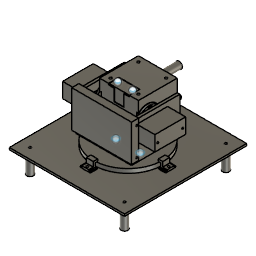
torretta_modulare_stampabile_v6_doppia_D_5x3x6 (Autodesk Fusion 360 design; units mm, degrees)
part number: 2026-07-14-16-52-52-233
part number: 2026-07-14-16-52-52-512
part number: 2026-07-14-16-52-55-927
part number: 2026-07-14-16-52-56-118
part number: 2026-07-14-16-52-56-486
part number: 2026-07-14-16-52-56-983
part number: 2026-07-14-16-52-59-861
part number: 2026-07-14-16-53-01-175
part number: 2026-07-14-16-53-03-719
part number: 2026-07-14-16-53-06-928
part number: 2026-07-14-16-53-10-286
part number: 2026-07-14-16-53-52-577
part number: 2026-07-14-16-53-58-816
part number: 2026-07-14-16-54-05-339
part number: 2026-07-14-16-54-28-797
part number: 2026-07-14-16-54-36-418
part number: 2026-07-14-16-54-44-458
part number: 2026-07-14-16-54-54-993
part number: 2026-07-14-16-55-05-930
part number: 2026-07-14-16-55-25-983
part number: 2026-07-14-16-55-55-201
part number: 2026-07-14-16-56-11-830
part number: 2026-07-14-16-56-28-975
part number: 2026-07-14-16-57-31-227
Autodesk Fusion 360 part; units mm, degrees
(part 1 of 3)
ref_plane "Piano di lavoro1" through (0, 0, 30) normal (0, 0, 1) x (1, 0, 0) in component "01_Tetto_elettronica_removibile"
sketch "Schizzo1" plane through (0, 0, 30) normal (0, 0, 1) x (1, 0, 0) in component "01_Tetto_elettronica_removibile"
  line L0 (-83, -88) -> (83, -88)
  line L1 (83, -88) -> (83, 88)
  line L2 (83, 88) -> (-83, 88)
  line L3 (-83, 88) -> (-83, -88)
extrude "Estrusione_Tetto_coperchio" add sketch "Schizzo1" along normal blind 3 makes body 1 in component "01_Tetto_elettronica_removibile"
sketch "Schizzo2" plane through (0, 0, 0) normal (0, 0, 1) x (1, 0, 0) in component "01_Tetto_elettronica_removibile"
  circle A0 centre (-68, -73) radius 5
extrude "Estrusione_Boss_verticale_M3_coperchio_01" add sketch "Schizzo2" along normal blind 33 bodies 1 in component "01_Tetto_elettronica_removibile"
sketch "Schizzo3" plane through (0, 0, 0) normal (0, 0, 1) x (1, 0, 0) in component "01_Tetto_elettronica_removibile"
  circle A0 centre (-68, -73) radius 1.6
extrude "Foro_M3_accessibile_dal_tetto_01" cut sketch "Schizzo3" along normal blind 33 bodies 1 in component "01_Tetto_elettronica_removibile"
sketch "Schizzo4" plane through (0, 0, 0) normal (0, 0, 1) x (1, 0, 0) in component "01_Tetto_elettronica_removibile"
  circle A0 centre (68, -73) radius 5
extrude "Estrusione_Boss_verticale_M3_coperchio_02" add sketch "Schizzo4" along normal blind 33 bodies 1 in component "01_Tetto_elettronica_removibile"
sketch "Schizzo5" plane through (0, 0, 0) normal (0, 0, 1) x (1, 0, 0) in component "01_Tetto_elettronica_removibile"
  circle A0 centre (68, -73) radius 1.6
extrude "Foro_M3_accessibile_dal_tetto_02" cut sketch "Schizzo5" along normal blind 33 bodies 1 in component "01_Tetto_elettronica_removibile"
sketch "Schizzo6" plane through (0, 0, 0) normal (0, 0, 1) x (1, 0, 0) in component "01_Tetto_elettronica_removibile"
  circle A0 centre (-68, 73) radius 5
extrude "Estrusione_Boss_verticale_M3_coperchio_03" add sketch "Schizzo6" along normal blind 33 bodies 1 in component "01_Tetto_elettronica_removibile"
sketch "Schizzo7" plane through (0, 0, 0) normal (0, 0, 1) x (1, 0, 0) in component "01_Tetto_elettronica_removibile"
  circle A0 centre (-68, 73) radius 1.6
extrude "Foro_M3_accessibile_dal_tetto_03" cut sketch "Schizzo7" along normal blind 33 bodies 1 in component "01_Tetto_elettronica_removibile"
sketch "Schizzo8" plane through (0, 0, 0) normal (0, 0, 1) x (1, 0, 0) in component "01_Tetto_elettronica_removibile"
  circle A0 centre (68, 73) radius 5
extrude "Estrusione_Boss_verticale_M3_coperchio_04" add sketch "Schizzo8" along normal blind 33 bodies 1 in component "01_Tetto_elettronica_removibile"
sketch "Schizzo9" plane through (0, 0, 0) normal (0, 0, 1) x (1, 0, 0) in component "01_Tetto_elettronica_removibile"
  circle A0 centre (68, 73) radius 1.6
extrude "Foro_M3_accessibile_dal_tetto_04" cut sketch "Schizzo9" along normal blind 33 bodies 1 in component "01_Tetto_elettronica_removibile"
ref_plane "Piano di lavoro2" through (0, 0, 30) normal (0, 0, 1) x (1, 0, 0) in component "01_Tetto_elettronica_removibile"
ref_plane "Piano di lavoro3" through (0, 0, 33) normal (0, 0, 1) x (1, 0, 0) in component "01_Tetto_elettronica_removibile"
ref_plane "Piano di lavoro4" through (0, 0, 30.9) normal (0, 0, 1) x (1, 0, 0) in component "01_Tetto_elettronica_removibile"
sketch "Schizzo10" plane through (0, 0, 30) normal (0, 0, 1) x (1, 0, 0) in component "01_Tetto_elettronica_removibile"
  circle A0 centre (0, 0) radius 6.25
extrude "Passaggio_albero_stepper" cut sketch "Schizzo10" along normal blind 3 bodies 1 in component "01_Tetto_elettronica_removibile"
sketch "Schizzo11" plane through (0, 0, 30) normal (0, 0, 1) x (1, 0, 0) in component "01_Tetto_elettronica_removibile"
  circle A0 centre (-17.5, 0) radius 2.1
extrude "Foro_stepper_Ovest" cut sketch "Schizzo11" along normal blind 3 bodies 1 in component "01_Tetto_elettronica_removibile"
sketch "Schizzo12" plane through (0, 0, 30.9) normal (0, 0, 1) x (1, 0, 0) in component "01_Tetto_elettronica_removibile"
  circle A0 centre (-17.5, 0) radius 2.1
sketch "Schizzo13" plane through (0, 0, 33) normal (0, 0, 1) x (1, 0, 0) in component "01_Tetto_elettronica_removibile"
  circle A0 centre (-17.5, 0) radius 4.2
loft "Svasatura_90_gradi_stepper_Ovest" cut profiles "Schizzo12", "Schizzo13" section 1 section 2 bodies 1 in component "01_Tetto_elettronica_removibile"
sketch "Schizzo14" plane through (0, 0, 30) normal (0, 0, 1) x (1, 0, 0) in component "01_Tetto_elettronica_removibile"
  circle A0 centre (17.5, 0) radius 2.1
extrude "Foro_stepper_Est" cut sketch "Schizzo14" along normal blind 3 bodies 1 in component "01_Tetto_elettronica_removibile"
sketch "Schizzo15" plane through (0, 0, 30.9) normal (0, 0, 1) x (1, 0, 0) in component "01_Tetto_elettronica_removibile"
  circle A0 centre (17.5, 0) radius 2.1
sketch "Schizzo16" plane through (0, 0, 33) normal (0, 0, 1) x (1, 0, 0) in component "01_Tetto_elettronica_removibile"
  circle A0 centre (17.5, 0) radius 4.2
loft "Svasatura_90_gradi_stepper_Est" cut profiles "Schizzo15", "Schizzo16" section 1 section 2 bodies 1 in component "01_Tetto_elettronica_removibile"
sketch "Schizzo17" plane through (0, 0, 30) normal (0, 0, 1) x (1, 0, 0) in component "01_Tetto_elettronica_removibile"
  circle A0 centre (58.5, 0) radius 1.6
extrude "Foro_M3_fermaglio_anti_sollevamento_Est" cut sketch "Schizzo17" along normal blind 3 bodies 1 in component "01_Tetto_elettronica_removibile"
sketch "Schizzo18" plane through (0, 0, 30) normal (0, 0, 1) x (1, 0, 0) in component "01_Tetto_elettronica_removibile"
  line L0 (61.4, 1.6743) -> (58.5, 3.3486)
  line L1 (58.5, 3.3486) -> (55.6, 1.6743)
  line L2 (55.6, 1.6743) -> (55.6, -1.6743)
  line L3 (55.6, -1.6743) -> (58.5, -3.3486)
  line L4 (58.5, -3.3486) -> (61.4, -1.6743)
  line L5 (61.4, -1.6743) -> (61.4, 1.6743)
extrude "Sede_dado_M3_fermaglio_Est" cut sketch "Schizzo18" along normal blind 2.6 bodies 1 in component "01_Tetto_elettronica_removibile"
sketch "Schizzo19" plane through (0, 0, 30) normal (0, 0, 1) x (1, 0, 0) in component "01_Tetto_elettronica_removibile"
  circle A0 centre (-58.5, 0) radius 1.6
extrude "Foro_M3_fermaglio_anti_sollevamento_Ovest" cut sketch "Schizzo19" along normal blind 3 bodies 1 in component "01_Tetto_elettronica_removibile"
sketch "Schizzo20" plane through (0, 0, 30) normal (0, 0, 1) x (1, 0, 0) in component "01_Tetto_elettronica_removibile"
  line L0 (-55.6, 1.6743) -> (-58.5, 3.3486)
  line L1 (-58.5, 3.3486) -> (-61.4, 1.6743)
  line L2 (-61.4, 1.6743) -> (-61.4, -1.6743)
  line L3 (-61.4, -1.6743) -> (-58.5, -3.3486)
  line L4 (-58.5, -3.3486) -> (-55.6, -1.6743)
  line L5 (-55.6, -1.6743) -> (-55.6, 1.6743)
extrude "Sede_dado_M3_fermaglio_Ovest" cut sketch "Schizzo20" along normal blind 2.6 bodies 1 in component "01_Tetto_elettronica_removibile"
sketch "Schizzo21" plane through (0, 0, 30) normal (0, 0, 1) x (1, 0, 0) in component "01_Tetto_elettronica_removibile"
  circle A0 centre (0, 58.5) radius 1.6
extrude "Foro_M3_fermaglio_anti_sollevamento_Nord" cut sketch "Schizzo21" along normal blind 3 bodies 1 in component "01_Tetto_elettronica_removibile"
sketch "Schizzo22" plane through (0, 0, 30) normal (0, 0, 1) x (1, 0, 0) in component "01_Tetto_elettronica_removibile"
  line L0 (2.9, 60.1743) -> (0, 61.8486)
  line L1 (0, 61.8486) -> (-2.9, 60.1743)
  line L2 (-2.9, 60.1743) -> (-2.9, 56.8257)
  line L3 (-2.9, 56.8257) -> (0, 55.1514)
  line L4 (0, 55.1514) -> (2.9, 56.8257)
  line L5 (2.9, 56.8257) -> (2.9, 60.1743)
extrude "Sede_dado_M3_fermaglio_Nord" cut sketch "Schizzo22" along normal blind 2.6 bodies 1 in component "01_Tetto_elettronica_removibile"
sketch "Schizzo23" plane through (0, 0, 30) normal (0, 0, 1) x (1, 0, 0) in component "01_Tetto_elettronica_removibile"
  circle A0 centre (0, -58.5) radius 1.6
extrude "Foro_M3_fermaglio_anti_sollevamento_Sud" cut sketch "Schizzo23" along normal blind 3 bodies 1 in component "01_Tetto_elettronica_removibile"
sketch "Schizzo24" plane through (0, 0, 30) normal (0, 0, 1) x (1, 0, 0) in component "01_Tetto_elettronica_removibile"
  line L0 (2.9, -56.8257) -> (0, -55.1514)
  line L1 (0, -55.1514) -> (-2.9, -56.8257)
  line L2 (-2.9, -56.8257) -> (-2.9, -60.1743)
  line L3 (-2.9, -60.1743) -> (0, -61.8486)
  line L4 (0, -61.8486) -> (2.9, -60.1743)
  line L5 (2.9, -60.1743) -> (2.9, -56.8257)
extrude "Sede_dado_M3_fermaglio_Sud" cut sketch "Schizzo24" along normal blind 2.6 bodies 1 in component "01_Tetto_elettronica_removibile"
ref_plane "Piano di lavoro5" through (0, 0, 22.8) normal (0, 0, 1) x (1, 0, 0) in component "01_Tetto_elettronica_removibile"
sketch "Schizzo25" plane through (0, 0, 22.8) normal (0, 0, 1) x (1, 0, 0) in component "01_Tetto_elettronica_removibile"
  circle A0 centre (0, 0) radius 23.5
  circle A1 centre (0, 0) radius 22
extrude "Estrusione_Parete_interna_liscia_canale_cavi" add sketch "Schizzo25" along normal blind 7.4 bodies 1 in component "01_Tetto_elettronica_removibile"
sketch "Schizzo26" plane through (0, 0, 22.8) normal (0, 0, 1) x (1, 0, 0) in component "01_Tetto_elettronica_removibile"
  circle A0 centre (0, 0) radius 34
  circle A1 centre (0, 0) radius 32.5
extrude "Estrusione_Parete_esterna_liscia_canale_cavi" add sketch "Schizzo26" along normal blind 7.4 bodies 1 in component "01_Tetto_elettronica_removibile"
ref_plane "Piano di lavoro6" through (0, 0, 20) normal (0, 0, 1) x (1, 0, 0) in component "01_Tetto_elettronica_removibile"
sketch "Schizzo27" plane through (0, 0, 20) normal (0, 0, 1) x (1, 0, 0) in component "01_Tetto_elettronica_removibile"
  circle A0 centre (0, 0) radius 40
  circle A1 centre (0, 0) radius 19
extrude "Estrusione_Fondo_anulare_continuo_canale_cavi" add sketch "Schizzo27" along normal blind 3 bodies 1 in component "01_Tetto_elettronica_removibile"
sketch "Schizzo28" plane through (0, 0, 20) normal (0, 0, 1) x (1, 0, 0) in component "01_Tetto_elettronica_removibile"
  line L0 (19.0919, 14.1421) -> (25.4558, 20.5061)
  line L1 (25.4558, 20.5061) -> (20.5061, 25.4558)
  line L2 (20.5061, 25.4558) -> (14.1421, 19.0919)
  line L3 (14.1421, 19.0919) -> (19.0919, 14.1421)
extrude "Uscita_fissa_9x7_canale_cavi_verso_vano_elettronica" cut sketch "Schizzo28" along normal blind 3 bodies 1 in component "01_Tetto_elettronica_removibile"
ref_plane "Piano di lavoro7" through (0, 0, 18) normal (0, 0, 1) x (1, 0, 0) in component "01_Tetto_elettronica_removibile"
sketch "Schizzo29" plane through (0, 0, 18) normal (0, 0, 1) x (1, 0, 0) in component "01_Tetto_elettronica_removibile"
  line L0 (23, 26) -> (41, 26)
  line L1 (41, 26) -> (41, 38)
  line L2 (41, 38) -> (23, 38)
  line L3 (23, 38) -> (23, 26)
extrude "Estrusione_Piastrina_fermacavo_fissa_sotto_uscita" add sketch "Schizzo29" along normal blind 2.2 bodies 1 in component "01_Tetto_elettronica_removibile"
sketch "Schizzo30" plane through (0, 0, 18) normal (0, 0, 1) x (1, 0, 0) in component "01_Tetto_elettronica_removibile"
  line L0 (7, 29) -> (27, 29)
  line L1 (27, 29) -> (27, 33)
  line L2 (27, 33) -> (7, 33)
  line L3 (7, 33) -> (7, 29)
extrude "Estrusione_Ponte_strutturale_fermacavo_fisso" add sketch "Schizzo30" along normal blind 2.2 bodies 1 in component "01_Tetto_elettronica_removibile"
sketch "Schizzo31" plane through (0, 0, 18) normal (0, 0, 1) x (1, 0, 0) in component "01_Tetto_elettronica_removibile"
  line L0 (31, 27.5) -> (36, 27.5)
  line L1 (36, 27.5) -> (36, 29.5)
  line L2 (36, 29.5) -> (31, 29.5)
  line L3 (31, 29.5) -> (31, 27.5)
extrude "Asola_fermacavo_fissa_inferiore_01" cut sketch "Schizzo31" along normal blind 2.2 bodies 1 in component "01_Tetto_elettronica_removibile"
sketch "Schizzo32" plane through (0, 0, 18) normal (0, 0, 1) x (1, 0, 0) in component "01_Tetto_elettronica_removibile"
  line L0 (31, 34.5) -> (36, 34.5)
  line L1 (36, 34.5) -> (36, 36.5)
  line L2 (36, 36.5) -> (31, 36.5)
  line L3 (31, 36.5) -> (31, 34.5)
extrude "Asola_fermacavo_fissa_inferiore_02" cut sketch "Schizzo32" along normal blind 2.2 bodies 1 in component "01_Tetto_elettronica_removibile"
sketch "Schizzo33" plane through (0, 0, 30) normal (0, 0, 1) x (1, 0, 0) in component "01_Tetto_elettronica_removibile"
  circle A0 centre (0, 0) radius 32.5
  circle A1 centre (0, 0) radius 23.5
extrude "Guida_anulare_cavi_azimut_meno180_piu180" cut sketch "Schizzo33" along normal blind 3 bodies 1 in component "01_Tetto_elettronica_removibile"
ref_plane "Piano di lavoro8" through (0, 0, 32.7) normal (0, 0, 1) x (1, 0, 0) in component "01_Tetto_elettronica_removibile"
sketch "Schizzo34" plane through (0, 0, 32.7) normal (0, 0, 1) x (1, 0, 0) in component "01_Tetto_elettronica_removibile"
  circle A0 centre (0, 0) radius 47.2
  circle A1 centre (0, 0) radius 37.8
extrude "Sede_ribassata_rondella_assiale" cut sketch "Schizzo34" along normal blind 0.3 bodies 1 in component "01_Tetto_elettronica_removibile"
ref_plane "Piano di lavoro9" through (0, 0, 32.5) normal (0, 0, 1) x (1, 0, 0) in component "01_Tetto_elettronica_removibile"
sketch "Schizzo35" plane through (0, 0, 32.5) normal (0, 0, 1) x (1, 0, 0) in component "01_Tetto_elettronica_removibile"
  circle A0 centre (0, 0) radius 36.5
  circle A1 centre (0, 0) radius 34.5
extrude "Estrusione_Labbro_fisso_centraggio_radiale_torretta" add sketch "Schizzo35" along normal blind 3.1 separate body makes body 2 in component "01_Tetto_elettronica_removibile"
combine "Unione_labbro_fisso_al_tetto" operation add target body 1 tool bodies 2 in component "01_Tetto_elettronica_removibile"
ref_plane "Piano di lavoro10" through (0, 0, 32.8) normal (0, 0, 1) x (1, 0, 0) in component "01_Tetto_elettronica_removibile"
sketch "Schizzo36" plane through (0, 0, 32.8) normal (0, 0, 1) x (1, 0, 0) in component "01_Tetto_elettronica_removibile"
  line L0 (51.5, -7.3) -> (61.5, -7.3)
  line L1 (61.5, -7.3) -> (61.5, -5.3)
  line L2 (61.5, -5.3) -> (51.5, -5.3)
  line L3 (51.5, -5.3) -> (51.5, -7.3)
extrude "Estrusione_Spallamento_antirotazione_Est_01" add sketch "Schizzo36" along normal blind 1.7 bodies 1 in component "01_Tetto_elettronica_removibile"
sketch "Schizzo37" plane through (0, 0, 32.8) normal (0, 0, 1) x (1, 0, 0) in component "01_Tetto_elettronica_removibile"
  line L0 (51.5, 5.3) -> (61.5, 5.3)
  line L1 (61.5, 5.3) -> (61.5, 7.3)
  line L2 (61.5, 7.3) -> (51.5, 7.3)
  line L3 (51.5, 7.3) -> (51.5, 5.3)
extrude "Estrusione_Spallamento_antirotazione_Est_02" add sketch "Schizzo37" along normal blind 1.7 bodies 1 in component "01_Tetto_elettronica_removibile"
sketch "Schizzo38" plane through (0, 0, 32.8) normal (0, 0, 1) x (1, 0, 0) in component "01_Tetto_elettronica_removibile"
  line L0 (-61.5, -7.3) -> (-51.5, -7.3)
  line L1 (-51.5, -7.3) -> (-51.5, -5.3)
  line L2 (-51.5, -5.3) -> (-61.5, -5.3)
  line L3 (-61.5, -5.3) -> (-61.5, -7.3)
extrude "Estrusione_Spallamento_antirotazione_Ovest_01" add sketch "Schizzo38" along normal blind 1.7 bodies 1 in component "01_Tetto_elettronica_removibile"
sketch "Schizzo39" plane through (0, 0, 32.8) normal (0, 0, 1) x (1, 0, 0) in component "01_Tetto_elettronica_removibile"
  line L0 (-61.5, 5.3) -> (-51.5, 5.3)
  line L1 (-51.5, 5.3) -> (-51.5, 7.3)
  line L2 (-51.5, 7.3) -> (-61.5, 7.3)
  line L3 (-61.5, 7.3) -> (-61.5, 5.3)
extrude "Estrusione_Spallamento_antirotazione_Ovest_02" add sketch "Schizzo39" along normal blind 1.7 bodies 1 in component "01_Tetto_elettronica_removibile"
sketch "Schizzo40" plane through (0, 0, 32.8) normal (0, 0, 1) x (1, 0, 0) in component "01_Tetto_elettronica_removibile"
  line L0 (-7.3, 51.5) -> (-5.3, 51.5)
  line L1 (-5.3, 51.5) -> (-5.3, 61.5)
  line L2 (-5.3, 61.5) -> (-7.3, 61.5)
  line L3 (-7.3, 61.5) -> (-7.3, 51.5)
extrude "Estrusione_Spallamento_antirotazione_Nord_01" add sketch "Schizzo40" along normal blind 1.7 bodies 1 in component "01_Tetto_elettronica_removibile"
sketch "Schizzo41" plane through (0, 0, 32.8) normal (0, 0, 1) x (1, 0, 0) in component "01_Tetto_elettronica_removibile"
  line L0 (5.3, 51.5) -> (7.3, 51.5)
  line L1 (7.3, 51.5) -> (7.3, 61.5)
  line L2 (7.3, 61.5) -> (5.3, 61.5)
  line L3 (5.3, 61.5) -> (5.3, 51.5)
extrude "Estrusione_Spallamento_antirotazione_Nord_02" add sketch "Schizzo41" along normal blind 1.7 bodies 1 in component "01_Tetto_elettronica_removibile"
sketch "Schizzo42" plane through (0, 0, 32.8) normal (0, 0, 1) x (1, 0, 0) in component "01_Tetto_elettronica_removibile"
  line L0 (-7.3, -61.5) -> (-5.3, -61.5)
  line L1 (-5.3, -61.5) -> (-5.3, -51.5)
  line L2 (-5.3, -51.5) -> (-7.3, -51.5)
  line L3 (-7.3, -51.5) -> (-7.3, -61.5)
extrude "Estrusione_Spallamento_antirotazione_Sud_01" add sketch "Schizzo42" along normal blind 1.7 bodies 1 in component "01_Tetto_elettronica_removibile"
sketch "Schizzo43" plane through (0, 0, 32.8) normal (0, 0, 1) x (1, 0, 0) in component "01_Tetto_elettronica_removibile"
  line L0 (5.3, -61.5) -> (7.3, -61.5)
  line L1 (7.3, -61.5) -> (7.3, -51.5)
  line L2 (7.3, -51.5) -> (5.3, -51.5)
  line L3 (5.3, -51.5) -> (5.3, -61.5)
extrude "Estrusione_Spallamento_antirotazione_Sud_02" add sketch "Schizzo43" along normal blind 1.7 bodies 1 in component "01_Tetto_elettronica_removibile"
ref_plane "Piano di lavoro1" through (0, 0, 32.7) normal (0, 0, 1) x (1, 0, 0) in component "02A_Rondella_assiale_torretta_sostituibile"
sketch "Schizzo1 (2)" plane through (0, 0, 32.7) normal (0, 0, 1) x (1, 0, 0) in component "02A_Rondella_assiale_torretta_sostituibile"
  circle A0 centre (0, 0) radius 47
  circle A1 centre (0, 0) radius 38
extrude "Estrusione_Rondella_assiale_basso_attrito" add sketch "Schizzo1 (2)" along normal blind 0.8 separate body makes body 3 in component "02A_Rondella_assiale_torretta_sostituibile"
ref_plane "Piano di lavoro1" through (0, 0, 10) normal (0, 0, 1) x (1, 0, 0) in component "02_Stepper_28BYJ48_statore_fisso_riferimento"
sketch "Schizzo1 (3)" plane through (0, 0, 10) normal (0, 0, 1) x (1, 0, 0) in component "02_Stepper_28BYJ48_statore_fisso_riferimento"
  circle A0 centre (0, 0) radius 14
extrude "Estrusione_Corpo_stepper" add sketch "Schizzo1 (3)" along normal blind 20 separate body makes body 4 in component "02_Stepper_28BYJ48_statore_fisso_riferimento"
ref_plane "Piano di lavoro2" through (0, 0, 27) normal (0, 0, 1) x (1, 0, 0) in component "02_Stepper_28BYJ48_statore_fisso_riferimento"
sketch "Schizzo2 (2)" plane through (0, 0, 27) normal (0, 0, 1) x (1, 0, 0) in component "02_Stepper_28BYJ48_statore_fisso_riferimento"
  line L0 (-20.75, -4) -> (20.75, -4)
  line L1 (20.75, -4) -> (20.75, 4)
  line L2 (20.75, 4) -> (-20.75, 4)
  line L3 (-20.75, 4) -> (-20.75, -4)
extrude "Estrusione_Alette_fissaggio_stepper" add sketch "Schizzo2 (2)" along normal blind 3 bodies 4 in component "02_Stepper_28BYJ48_statore_fisso_riferimento"
ref_plane "Piano di lavoro1" through (0, 0, 30) normal (0, 0, 1) x (1, 0, 0) in component "02B_Rotore_albero_28BYJ48_riferimento"
sketch "Schizzo1 (4)" plane through (0, 0, 30) normal (0, 0, 1) x (1, 0, 0) in component "02B_Rotore_albero_28BYJ48_riferimento"
  circle A0 centre (0, 0) radius 2.5
extrude "Estrusione_Albero_stepper" add sketch "Schizzo1 (4)" along normal blind 6 separate body makes body 5 in component "02B_Rotore_albero_28BYJ48_riferimento"
sketch "Schizzo2 (3)" plane through (0, 0, 30) normal (0, 0, 1) x (1, 0, 0) in component "02B_Rotore_albero_28BYJ48_riferimento"
  line L0 (-2.5, -2.7) -> (-1.5, -2.7)
  line L1 (-1.5, -2.7) -> (-1.5, 2.7)
  line L2 (-1.5, 2.7) -> (-2.5, 2.7)
  line L3 (-2.5, 2.7) -> (-2.5, -2.7)
extrude "Piatto_sinistro_albero_stepper" cut sketch "Schizzo2 (3)" along normal blind 6 bodies 5 in component "02B_Rotore_albero_28BYJ48_riferimento"
sketch "Schizzo3 (2)" plane through (0, 0, 30) normal (0, 0, 1) x (1, 0, 0) in component "02B_Rotore_albero_28BYJ48_riferimento"
  line L0 (1.5, -2.7) -> (2.5, -2.7)
  line L1 (2.5, -2.7) -> (2.5, 2.7)
  line L2 (2.5, 2.7) -> (1.5, 2.7)
  line L3 (1.5, 2.7) -> (1.5, -2.7)
extrude "Piatto_destro_albero_stepper" cut sketch "Schizzo3 (2)" along normal blind 6 bodies 5 in component "02B_Rotore_albero_28BYJ48_riferimento"
ref_plane "Piano di lavoro1" through (0, 0, 33.5) normal (0, 0, 1) x (1, 0, 0) in component "03_Base_rotante_D100_sede_D_stepper"
sketch "Schizzo1 (5)" plane through (0, 0, 33.5) normal (0, 0, 1) x (1, 0, 0) in component "03_Base_rotante_D100_sede_D_stepper"
  circle A0 centre (0, 0) radius 50
extrude "Estrusione_Piastra_base_rotante_D100" add sketch "Schizzo1 (5)" along normal blind 6 separate body makes body 6 in component "03_Base_rotante_D100_sede_D_stepper"
ref_plane "Piano di lavoro2" through (0, 0, 31.5) normal (0, 0, 1) x (1, 0, 0) in component "03_Base_rotante_D100_sede_D_stepper"
sketch "Schizzo2 (4)" plane through (0, 0, 31.5) normal (0, 0, 1) x (1, 0, 0) in component "03_Base_rotante_D100_sede_D_stepper"
  circle A0 centre (0, 0) radius 6
extrude "Estrusione_Mozzo_inferiore_accoppiamento_stepper" add sketch "Schizzo2 (4)" along normal blind 2.2 bodies 6 in component "03_Base_rotante_D100_sede_D_stepper"
sketch "Schizzo3 (3)" plane through (0, 0, 31.5) normal (0, 0, 1) x (1, 0, 0) in component "03_Base_rotante_D100_sede_D_stepper"
  circle A0 centre (0, 0) radius 2.7
extrude "Preforo_circolare_sede_D_stepper" cut sketch "Schizzo3 (3)" along normal blind 8.2 bodies 5 in component "02B_Rotore_albero_28BYJ48_riferimento"
extrude "Estrusione3" cut sketch "Schizzo3 (3)" along normal blind 8.2 bodies 6 in component "03_Base_rotante_D100_sede_D_stepper"
sketch "Schizzo4 (2)" plane through (0, 0, 33.5) normal (0, 0, 1) x (1, 0, 0) in component "03_Base_rotante_D100_sede_D_stepper"
  line L0 (-2.7, -2.9) -> (-1.7, -2.9)
  line L1 (-1.7, -2.9) -> (-1.7, 2.9)
  line L2 (-1.7, 2.9) -> (-2.7, 2.9)
  line L3 (-2.7, 2.9) -> (-2.7, -2.9)
extrude "Estrusione_Riempimento_lato_sinistro_sede_doppia_D" add sketch "Schizzo4 (2)" along normal blind 8.2 bodies 6 in component "03_Base_rotante_D100_sede_D_stepper"
sketch "Schizzo5 (2)" plane through (0, 0, 33.5) normal (0, 0, 1) x (1, 0, 0) in component "03_Base_rotante_D100_sede_D_stepper"
  line L0 (1.7, -2.9) -> (2.7, -2.9)
  line L1 (2.7, -2.9) -> (2.7, 2.9)
  line L2 (2.7, 2.9) -> (1.7, 2.9)
  line L3 (1.7, 2.9) -> (1.7, -2.9)
extrude "Estrusione_Riempimento_lato_destro_sede_doppia_D" add sketch "Schizzo5 (2)" along normal blind 8.2 bodies 6 in component "03_Base_rotante_D100_sede_D_stepper"
sketch "Schizzo6 (2)" plane through (0, 0, 33.5) normal (0, 0, 1) x (1, 0, 0) in component "03_Base_rotante_D100_sede_D_stepper"
  circle A0 centre (0, 0) radius 36.8
  circle A1 centre (0, 0) radius 34.2
extrude "Gola_inferiore_centraggio_radiale_con_gioco" cut sketch "Schizzo6 (2)" along normal blind 2.5 bodies 1 in component "01_Tetto_elettronica_removibile"
extrude "Estrusione6" cut sketch "Schizzo6 (2)" along normal blind 2.5 bodies 6 in component "03_Base_rotante_D100_sede_D_stepper"
ref_plane "Piano di lavoro3" through (0, 0, 36.9) normal (0, 0, 1) x (1, 0, 0) in component "03_Base_rotante_D100_sede_D_stepper"
sketch "Schizzo7 (2)" plane through (0, 0, 33.5) normal (0, 0, 1) x (1, 0, 0) in component "03_Base_rotante_D100_sede_D_stepper"
  circle A0 centre (-19, 0) radius 1.6
extrude "Foro_M3_adattatore_01" cut sketch "Schizzo7 (2)" along normal blind 6 bodies 6 in component "03_Base_rotante_D100_sede_D_stepper"
sketch "Schizzo8 (2)" plane through (0, 0, 36.9) normal (0, 0, 1) x (1, 0, 0) in component "03_Base_rotante_D100_sede_D_stepper"
  line L0 (-16.1, 1.6743) -> (-19, 3.3486)
  line L1 (-19, 3.3486) -> (-21.9, 1.6743)
  line L2 (-21.9, 1.6743) -> (-21.9, -1.6743)
  line L3 (-21.9, -1.6743) -> (-19, -3.3486)
  line L4 (-19, -3.3486) -> (-16.1, -1.6743)
  line L5 (-16.1, -1.6743) -> (-16.1, 1.6743)
extrude "Sede_dado_M3_adattatore_01" cut sketch "Schizzo8 (2)" along normal blind 2.6 bodies 6 in component "03_Base_rotante_D100_sede_D_stepper"
sketch "Schizzo9 (2)" plane through (0, 0, 33.5) normal (0, 0, 1) x (1, 0, 0) in component "03_Base_rotante_D100_sede_D_stepper"
  circle A0 centre (19, 0) radius 1.6
extrude "Foro_M3_adattatore_02" cut sketch "Schizzo9 (2)" along normal blind 6 bodies 6 in component "03_Base_rotante_D100_sede_D_stepper"
sketch "Schizzo10 (2)" plane through (0, 0, 36.9) normal (0, 0, 1) x (1, 0, 0) in component "03_Base_rotante_D100_sede_D_stepper"
  line L0 (21.9, 1.6743) -> (19, 3.3486)
  line L1 (19, 3.3486) -> (16.1, 1.6743)
  line L2 (16.1, 1.6743) -> (16.1, -1.6743)
  line L3 (16.1, -1.6743) -> (19, -3.3486)
  line L4 (19, -3.3486) -> (21.9, -1.6743)
  line L5 (21.9, -1.6743) -> (21.9, 1.6743)
extrude "Sede_dado_M3_adattatore_02" cut sketch "Schizzo10 (2)" along normal blind 2.6 bodies 6 in component "03_Base_rotante_D100_sede_D_stepper"
sketch "Schizzo11 (2)" plane through (0, 0, 33.5) normal (0, 0, 1) x (1, 0, 0) in component "03_Base_rotante_D100_sede_D_stepper"
  circle A0 centre (0, -19) radius 1.6
extrude "Foro_M3_adattatore_03" cut sketch "Schizzo11 (2)" along normal blind 6 bodies 6 in component "03_Base_rotante_D100_sede_D_stepper"
sketch "Schizzo12 (2)" plane through (0, 0, 36.9) normal (0, 0, 1) x (1, 0, 0) in component "03_Base_rotante_D100_sede_D_stepper"
  line L0 (2.9, -17.3257) -> (0, -15.6514)
  line L1 (0, -15.6514) -> (-2.9, -17.3257)
  line L2 (-2.9, -17.3257) -> (-2.9, -20.6743)
  line L3 (-2.9, -20.6743) -> (0, -22.3486)
  line L4 (0, -22.3486) -> (2.9, -20.6743)
  line L5 (2.9, -20.6743) -> (2.9, -17.3257)
extrude "Sede_dado_M3_adattatore_03" cut sketch "Schizzo12 (2)" along normal blind 2.6 bodies 6 in component "03_Base_rotante_D100_sede_D_stepper"
sketch "Schizzo13 (2)" plane through (0, 0, 33.5) normal (0, 0, 1) x (1, 0, 0) in component "03_Base_rotante_D100_sede_D_stepper"
  circle A0 centre (0, 19) radius 1.6
extrude "Foro_M3_adattatore_04" cut sketch "Schizzo13 (2)" along normal blind 6 bodies 6 in component "03_Base_rotante_D100_sede_D_stepper"
sketch "Schizzo14 (2)" plane through (0, 0, 36.9) normal (0, 0, 1) x (1, 0, 0) in component "03_Base_rotante_D100_sede_D_stepper"
  line L0 (2.9, 20.6743) -> (0, 22.3486)
  line L1 (0, 22.3486) -> (-2.9, 20.6743)
  line L2 (-2.9, 20.6743) -> (-2.9, 17.3257)
  line L3 (-2.9, 17.3257) -> (0, 15.6514)
  line L4 (0, 15.6514) -> (2.9, 17.3257)
  line L5 (2.9, 17.3257) -> (2.9, 20.6743)
extrude "Sede_dado_M3_adattatore_04" cut sketch "Schizzo14 (2)" along normal blind 2.6 bodies 6 in component "03_Base_rotante_D100_sede_D_stepper"
sketch "Schizzo15 (2)" plane through (0, 0, 33.5) normal (0, 0, 1) x (1, 0, 0) in component "03_Base_rotante_D100_sede_D_stepper"
  line L0 (19.0919, 14.1421) -> (25.4558, 20.5061)
  line L1 (25.4558, 20.5061) -> (20.5061, 25.4558)
  line L2 (20.5061, 25.4558) -> (14.1421, 19.0919)
  line L3 (14.1421, 19.0919) -> (19.0919, 14.1421)
extrude "Passaggio_9x7_comune_servi_cannone_adattatore" cut sketch "Schizzo15 (2)" along normal blind 6 bodies 6 in component "03_Base_rotante_D100_sede_D_stepper"
ref_plane "Piano di lavoro1" through (0, 0, 33) normal (0, 0, 1) x (1, 0, 0) in component "03A_Fermaglio_anti_sollevamento_Est_M3"
ref_plane "Piano di lavoro2" through (0, 0, 36) normal (0, 0, 1) x (1, 0, 0) in component "03A_Fermaglio_anti_sollevamento_Est_M3"
ref_plane "Piano di lavoro3" through (0, 0, 39.9) normal (0, 0, 1) x (1, 0, 0) in component "03A_Fermaglio_anti_sollevamento_Est_M3"
sketch "Schizzo1 (6)" plane through (0, 0, 33) normal (0, 0, 1) x (1, 0, 0) in component "03A_Fermaglio_anti_sollevamento_Est_M3"
  line L0 (51.5, -5) -> (61.5, -5)
  line L1 (61.5, -5) -> (61.5, 5)
  line L2 (61.5, 5) -> (51.5, 5)
  line L3 (51.5, 5) -> (51.5, -5)
extrude "Estrusione_Piede_fermaglio_Est" add sketch "Schizzo1 (6)" along normal blind 3 separate body makes body 7 in component "03A_Fermaglio_anti_sollevamento_Est_M3"
sketch "Schizzo2 (5)" plane through (0, 0, 36) normal (0, 0, 1) x (1, 0, 0) in component "03A_Fermaglio_anti_sollevamento_Est_M3"
  line L0 (52, -5) -> (55, -5)
  line L1 (55, -5) -> (55, 5)
  line L2 (55, 5) -> (52, 5)
  line L3 (52, 5) -> (52, -5)
extrude "Estrusione_Montante_fermaglio_Est" add sketch "Schizzo2 (5)" along normal blind 3.9 bodies 7 in component "03A_Fermaglio_anti_sollevamento_Est_M3"
sketch "Schizzo3 (4)" plane through (0, 0, 39.9) normal (0, 0, 1) x (1, 0, 0) in component "03A_Fermaglio_anti_sollevamento_Est_M3"
  line L0 (48.5, -5) -> (55, -5)
  line L1 (55, -5) -> (55, 5)
  line L2 (55, 5) -> (48.5, 5)
  line L3 (48.5, 5) -> (48.5, -5)
extrude "Estrusione_Linguetta_fermaglio_Est" add sketch "Schizzo3 (4)" along normal blind 3 bodies 7 in component "03A_Fermaglio_anti_sollevamento_Est_M3"
sketch "Schizzo4 (3)" plane through (0, 0, 33) normal (0, 0, 1) x (1, 0, 0) in component "03A_Fermaglio_anti_sollevamento_Est_M3"
  circle A0 centre (58.5, 0) radius 1.6
extrude "Foro_M3_fermaglio_Est" cut sketch "Schizzo4 (3)" along normal blind 3 bodies 7 in component "03A_Fermaglio_anti_sollevamento_Est_M3"
ref_plane "Piano di lavoro1" through (0, 0, 33) normal (0, 0, 1) x (1, 0, 0) in component "03A_Fermaglio_anti_sollevamento_Ovest_M3"
ref_plane "Piano di lavoro2" through (0, 0, 36) normal (0, 0, 1) x (1, 0, 0) in component "03A_Fermaglio_anti_sollevamento_Ovest_M3"
ref_plane "Piano di lavoro3" through (0, 0, 39.9) normal (0, 0, 1) x (1, 0, 0) in component "03A_Fermaglio_anti_sollevamento_Ovest_M3"
sketch "Schizzo1 (7)" plane through (0, 0, 33) normal (0, 0, 1) x (1, 0, 0) in component "03A_Fermaglio_anti_sollevamento_Ovest_M3"
  line L0 (-61.5, -5) -> (-51.5, -5)
  line L1 (-51.5, -5) -> (-51.5, 5)
  line L2 (-51.5, 5) -> (-61.5, 5)
  line L3 (-61.5, 5) -> (-61.5, -5)
extrude "Estrusione_Piede_fermaglio_Ovest" add sketch "Schizzo1 (7)" along normal blind 3 separate body makes body 8 in component "03A_Fermaglio_anti_sollevamento_Ovest_M3"
sketch "Schizzo2 (6)" plane through (0, 0, 36) normal (0, 0, 1) x (1, 0, 0) in component "03A_Fermaglio_anti_sollevamento_Ovest_M3"
  line L0 (-55, -5) -> (-52, -5)
  line L1 (-52, -5) -> (-52, 5)
  line L2 (-52, 5) -> (-55, 5)
  line L3 (-55, 5) -> (-55, -5)
extrude "Estrusione_Montante_fermaglio_Ovest" add sketch "Schizzo2 (6)" along normal blind 3.9 bodies 8 in component "03A_Fermaglio_anti_sollevamento_Ovest_M3"
sketch "Schizzo3 (5)" plane through (0, 0, 39.9) normal (0, 0, 1) x (1, 0, 0) in component "03A_Fermaglio_anti_sollevamento_Ovest_M3"
  line L0 (-55, -5) -> (-48.5, -5)
  line L1 (-48.5, -5) -> (-48.5, 5)
  line L2 (-48.5, 5) -> (-55, 5)
  line L3 (-55, 5) -> (-55, -5)
extrude "Estrusione_Linguetta_fermaglio_Ovest" add sketch "Schizzo3 (5)" along normal blind 3 bodies 8 in component "03A_Fermaglio_anti_sollevamento_Ovest_M3"
sketch "Schizzo4 (4)" plane through (0, 0, 33) normal (0, 0, 1) x (1, 0, 0) in component "03A_Fermaglio_anti_sollevamento_Ovest_M3"
  circle A0 centre (-58.5, 0) radius 1.6
extrude "Foro_M3_fermaglio_Ovest" cut sketch "Schizzo4 (4)" along normal blind 3 bodies 8 in component "03A_Fermaglio_anti_sollevamento_Ovest_M3"
ref_plane "Piano di lavoro1" through (0, 0, 33) normal (0, 0, 1) x (1, 0, 0) in component "03A_Fermaglio_anti_sollevamento_Nord_M3"
ref_plane "Piano di lavoro2" through (0, 0, 36) normal (0, 0, 1) x (1, 0, 0) in component "03A_Fermaglio_anti_sollevamento_Nord_M3"
ref_plane "Piano di lavoro3" through (0, 0, 39.9) normal (0, 0, 1) x (1, 0, 0) in component "03A_Fermaglio_anti_sollevamento_Nord_M3"
sketch "Schizzo1 (8)" plane through (0, 0, 33) normal (0, 0, 1) x (1, 0, 0) in component "03A_Fermaglio_anti_sollevamento_Nord_M3"
  line L0 (-5, 51.5) -> (5, 51.5)
  line L1 (5, 51.5) -> (5, 61.5)
  line L2 (5, 61.5) -> (-5, 61.5)
  line L3 (-5, 61.5) -> (-5, 51.5)
extrude "Estrusione_Piede_fermaglio_Nord" add sketch "Schizzo1 (8)" along normal blind 3 separate body makes body 9 in component "03A_Fermaglio_anti_sollevamento_Nord_M3"
sketch "Schizzo2 (7)" plane through (0, 0, 36) normal (0, 0, 1) x (1, 0, 0) in component "03A_Fermaglio_anti_sollevamento_Nord_M3"
  line L0 (-5, 52) -> (5, 52)
  line L1 (5, 52) -> (5, 55)
  line L2 (5, 55) -> (-5, 55)
  line L3 (-5, 55) -> (-5, 52)
extrude "Estrusione_Montante_fermaglio_Nord" add sketch "Schizzo2 (7)" along normal blind 3.9 bodies 9 in component "03A_Fermaglio_anti_sollevamento_Nord_M3"
sketch "Schizzo3 (6)" plane through (0, 0, 39.9) normal (0, 0, 1) x (1, 0, 0) in component "03A_Fermaglio_anti_sollevamento_Nord_M3"
  line L0 (-5, 48.5) -> (5, 48.5)
  line L1 (5, 48.5) -> (5, 55)
  line L2 (5, 55) -> (-5, 55)
  line L3 (-5, 55) -> (-5, 48.5)
extrude "Estrusione_Linguetta_fermaglio_Nord" add sketch "Schizzo3 (6)" along normal blind 3 bodies 9 in component "03A_Fermaglio_anti_sollevamento_Nord_M3"
sketch "Schizzo4 (5)" plane through (0, 0, 33) normal (0, 0, 1) x (1, 0, 0) in component "03A_Fermaglio_anti_sollevamento_Nord_M3"
  circle A0 centre (0, 58.5) radius 1.6
extrude "Foro_M3_fermaglio_Nord" cut sketch "Schizzo4 (5)" along normal blind 3 bodies 9 in component "03A_Fermaglio_anti_sollevamento_Nord_M3"
ref_plane "Piano di lavoro1" through (0, 0, 33) normal (0, 0, 1) x (1, 0, 0) in component "03A_Fermaglio_anti_sollevamento_Sud_M3"
ref_plane "Piano di lavoro2" through (0, 0, 36) normal (0, 0, 1) x (1, 0, 0) in component "03A_Fermaglio_anti_sollevamento_Sud_M3"
ref_plane "Piano di lavoro3" through (0, 0, 39.9) normal (0, 0, 1) x (1, 0, 0) in component "03A_Fermaglio_anti_sollevamento_Sud_M3"
sketch "Schizzo1 (9)" plane through (0, 0, 33) normal (0, 0, 1) x (1, 0, 0) in component "03A_Fermaglio_anti_sollevamento_Sud_M3"
  line L0 (-5, -61.5) -> (5, -61.5)
  line L1 (5, -61.5) -> (5, -51.5)
  line L2 (5, -51.5) -> (-5, -51.5)
  line L3 (-5, -51.5) -> (-5, -61.5)
extrude "Estrusione_Piede_fermaglio_Sud" add sketch "Schizzo1 (9)" along normal blind 3 separate body makes body 10 in component "03A_Fermaglio_anti_sollevamento_Sud_M3"
sketch "Schizzo2 (8)" plane through (0, 0, 36) normal (0, 0, 1) x (1, 0, 0) in component "03A_Fermaglio_anti_sollevamento_Sud_M3"
  line L0 (-5, -55) -> (5, -55)
  line L1 (5, -55) -> (5, -52)
  line L2 (5, -52) -> (-5, -52)
  line L3 (-5, -52) -> (-5, -55)
extrude "Estrusione_Montante_fermaglio_Sud" add sketch "Schizzo2 (8)" along normal blind 3.9 bodies 10 in component "03A_Fermaglio_anti_sollevamento_Sud_M3"
sketch "Schizzo3 (7)" plane through (0, 0, 39.9) normal (0, 0, 1) x (1, 0, 0) in component "03A_Fermaglio_anti_sollevamento_Sud_M3"
  line L0 (-5, -55) -> (5, -55)
  line L1 (5, -55) -> (5, -48.5)
  line L2 (5, -48.5) -> (-5, -48.5)
  line L3 (-5, -48.5) -> (-5, -55)
extrude "Estrusione_Linguetta_fermaglio_Sud" add sketch "Schizzo3 (7)" along normal blind 3 bodies 10 in component "03A_Fermaglio_anti_sollevamento_Sud_M3"
sketch "Schizzo4 (6)" plane through (0, 0, 33) normal (0, 0, 1) x (1, 0, 0) in component "03A_Fermaglio_anti_sollevamento_Sud_M3"
  circle A0 centre (0, -58.5) radius 1.6
extrude "Foro_M3_fermaglio_Sud" cut sketch "Schizzo4 (6)" along normal blind 3 bodies 10 in component "03A_Fermaglio_anti_sollevamento_Sud_M3"
ref_plane "Piano di lavoro1" through (0, 0, 45.5) normal (0, 0, 1) x (1, 0, 0) in component "04_Torretta_parte_fissa_azimut"
sketch "Schizzo1 (10)" plane through (0, 0, 45.5) normal (0, 0, 1) x (1, 0, 0) in component "04_Torretta_parte_fissa_azimut"
  line L0 (-40, -35) -> (40, -35)
  line L1 (40, -35) -> (40, 35)
  line L2 (40, 35) -> (-40, 35)
  line L3 (-40, 35) -> (-40, -35)
extrude "Estrusione_Base_parte_fissa" add sketch "Schizzo1 (10)" along normal blind 4 separate body makes body 11 in component "04_Torretta_parte_fissa_azimut"
ref_plane "Piano di lavoro2" through (0, 0, 39.5) normal (0, 0, 1) x (1, 0, 0) in component "04_Torretta_parte_fissa_azimut"
sketch "Schizzo2 (9)" plane through (0, 0, 39.5) normal (0, 0, 1) x (1, 0, 0) in component "04_Torretta_parte_fissa_azimut"
  circle A0 centre (-19, 0) radius 5
extrude "Estrusione_Distanziale_telaio_M3_01" add sketch "Schizzo2 (9)" along normal blind 6.2 bodies 11 in component "04_Torretta_parte_fissa_azimut"
sketch "Schizzo3 (8)" plane through (0, 0, 39.5) normal (0, 0, 1) x (1, 0, 0) in component "04_Torretta_parte_fissa_azimut"
  circle A0 centre (-19, 0) radius 1.6
extrude "Foro_M3_base_fissa_01" cut sketch "Schizzo3 (8)" along normal blind 10 bodies 11 in component "04_Torretta_parte_fissa_azimut"
sketch "Schizzo4 (7)" plane through (0, 0, 39.5) normal (0, 0, 1) x (1, 0, 0) in component "04_Torretta_parte_fissa_azimut"
  circle A0 centre (19, 0) radius 5
extrude "Estrusione_Distanziale_telaio_M3_02" add sketch "Schizzo4 (7)" along normal blind 6.2 bodies 11 in component "04_Torretta_parte_fissa_azimut"
sketch "Schizzo5 (3)" plane through (0, 0, 39.5) normal (0, 0, 1) x (1, 0, 0) in component "04_Torretta_parte_fissa_azimut"
  circle A0 centre (19, 0) radius 1.6
extrude "Foro_M3_base_fissa_02" cut sketch "Schizzo5 (3)" along normal blind 10 bodies 11 in component "04_Torretta_parte_fissa_azimut"
sketch "Schizzo6 (3)" plane through (0, 0, 39.5) normal (0, 0, 1) x (1, 0, 0) in component "04_Torretta_parte_fissa_azimut"
  circle A0 centre (0, -19) radius 5
extrude "Estrusione_Distanziale_telaio_M3_03" add sketch "Schizzo6 (3)" along normal blind 6.2 bodies 11 in component "04_Torretta_parte_fissa_azimut"
sketch "Schizzo7 (3)" plane through (0, 0, 39.5) normal (0, 0, 1) x (1, 0, 0) in component "04_Torretta_parte_fissa_azimut"
  circle A0 centre (0, -19) radius 1.6
extrude "Foro_M3_base_fissa_03" cut sketch "Schizzo7 (3)" along normal blind 10 bodies 11 in component "04_Torretta_parte_fissa_azimut"
sketch "Schizzo8 (3)" plane through (0, 0, 39.5) normal (0, 0, 1) x (1, 0, 0) in component "04_Torretta_parte_fissa_azimut"
  circle A0 centre (0, 19) radius 5
extrude "Estrusione_Distanziale_telaio_M3_04" add sketch "Schizzo8 (3)" along normal blind 6.2 bodies 11 in component "04_Torretta_parte_fissa_azimut"
sketch "Schizzo9 (3)" plane through (0, 0, 39.5) normal (0, 0, 1) x (1, 0, 0) in component "04_Torretta_parte_fissa_azimut"
  circle A0 centre (0, 19) radius 1.6
extrude "Foro_M3_base_fissa_04" cut sketch "Schizzo9 (3)" along normal blind 10 bodies 11 in component "04_Torretta_parte_fissa_azimut"
sketch "Schizzo10 (3)" plane through (0, 0, 45.5) normal (0, 0, 1) x (1, 0, 0) in component "04_Torretta_parte_fissa_azimut"
  line L0 (19.0919, 14.1421) -> (25.4558, 20.5061)
  line L1 (25.4558, 20.5061) -> (20.5061, 25.4558)
  line L2 (20.5061, 25.4558) -> (14.1421, 19.0919)
  line L3 (14.1421, 19.0919) -> (19.0919, 14.1421)
extrude "Passaggio_9x7_comune_servi_cannone_base_fissa" cut sketch "Schizzo10 (3)" along normal blind 4 bodies 11 in component "04_Torretta_parte_fissa_azimut"
sketch "Schizzo11 (3)" plane through (0, 0, 45.5) normal (0, 0, 1) x (1, 0, 0) in component "04_Torretta_parte_fissa_azimut"
  line L0 (-30.5, -19.5) -> (-25.5, -19.5)
  line L1 (-25.5, -19.5) -> (-25.5, -17.5)
  line L2 (-25.5, -17.5) -> (-30.5, -17.5)
  line L3 (-30.5, -17.5) -> (-30.5, -19.5)
extrude "Asola_fermacavo_Servo_sinistro_01" cut sketch "Schizzo11 (3)" along normal blind 4 bodies 11 in component "04_Torretta_parte_fissa_azimut"
sketch "Schizzo12 (3)" plane through (0, 0, 45.5) normal (0, 0, 1) x (1, 0, 0) in component "04_Torretta_parte_fissa_azimut"
  line L0 (-30.5, -12.5) -> (-25.5, -12.5)
  line L1 (-25.5, -12.5) -> (-25.5, -10.5)
  line L2 (-25.5, -10.5) -> (-30.5, -10.5)
  line L3 (-30.5, -10.5) -> (-30.5, -12.5)
extrude "Asola_fermacavo_Servo_sinistro_02" cut sketch "Schizzo12 (3)" along normal blind 4 bodies 11 in component "04_Torretta_parte_fissa_azimut"
sketch "Schizzo13 (3)" plane through (0, 0, 45.5) normal (0, 0, 1) x (1, 0, 0) in component "04_Torretta_parte_fissa_azimut"
  line L0 (-2.5, -11.5) -> (2.5, -11.5)
  line L1 (2.5, -11.5) -> (2.5, -9.5)
  line L2 (2.5, -9.5) -> (-2.5, -9.5)
  line L3 (-2.5, -9.5) -> (-2.5, -11.5)
extrude "Asola_fermacavo_Cannone_01" cut sketch "Schizzo13 (3)" along normal blind 4 bodies 11 in component "04_Torretta_parte_fissa_azimut"
sketch "Schizzo14 (3)" plane through (0, 0, 45.5) normal (0, 0, 1) x (1, 0, 0) in component "04_Torretta_parte_fissa_azimut"
  line L0 (-2.5, -4.5) -> (2.5, -4.5)
  line L1 (2.5, -4.5) -> (2.5, -2.5)
  line L2 (2.5, -2.5) -> (-2.5, -2.5)
  line L3 (-2.5, -2.5) -> (-2.5, -4.5)
extrude "Asola_fermacavo_Cannone_02" cut sketch "Schizzo14 (3)" along normal blind 4 bodies 11 in component "04_Torretta_parte_fissa_azimut"
sketch "Schizzo15 (3)" plane through (0, 0, 45.5) normal (0, 0, 1) x (1, 0, 0) in component "04_Torretta_parte_fissa_azimut"
  line L0 (25.5, -19.5) -> (30.5, -19.5)
  line L1 (30.5, -19.5) -> (30.5, -17.5)
  line L2 (30.5, -17.5) -> (25.5, -17.5)
  line L3 (25.5, -17.5) -> (25.5, -19.5)
extrude "Asola_fermacavo_Servo_destro_01" cut sketch "Schizzo15 (3)" along normal blind 4 bodies 11 in component "04_Torretta_parte_fissa_azimut"
sketch "Schizzo16 (2)" plane through (0, 0, 45.5) normal (0, 0, 1) x (1, 0, 0) in component "04_Torretta_parte_fissa_azimut"
  line L0 (25.5, -12.5) -> (30.5, -12.5)
  line L1 (30.5, -12.5) -> (30.5, -10.5)
  line L2 (30.5, -10.5) -> (25.5, -10.5)
  line L3 (25.5, -10.5) -> (25.5, -12.5)
extrude "Asola_fermacavo_Servo_destro_02" cut sketch "Schizzo16 (2)" along normal blind 4 bodies 11 in component "04_Torretta_parte_fissa_azimut"
ref_plane "Piano di lavoro3" through (-40, 0, 0) normal (1, 0, 0) x (0, 1, 0) in component "04_Torretta_parte_fissa_azimut"
sketch "Schizzo17 (2)" plane through (-40, 0, 0) normal (1, 0, 0) x (0, 0, -1) in component "04_Torretta_parte_fissa_azimut"
  line L0 (-49.5, -35) -> (-99.5, -35)
  line L1 (-99.5, -35) -> (-99.5, 35)
  line L2 (-99.5, 35) -> (-49.5, 35)
  line L3 (-49.5, 35) -> (-49.5, -35)
extrude "Estrusione_Parete_fissa_Sinistra" add sketch "Schizzo17 (2)" along normal blind 4 bodies 11 in component "04_Torretta_parte_fissa_azimut"
ref_plane "Piano di lavoro4" through (-40, 0, 0) normal (1, 0, 0) x (0, 1, 0) in component "04_Torretta_parte_fissa_azimut"
sketch "Schizzo18 (2)" plane through (-40, 0, 0) normal (1, 0, 0) x (0, 0, -1) in component "04_Torretta_parte_fissa_azimut"
  line L0 (-74.9, -17.5) -> (-88.1, -17.5)
  line L1 (-88.1, -17.5) -> (-88.1, 6.2)
  line L2 (-88.1, 6.2) -> (-74.9, 6.2)
  line L3 (-74.9, 6.2) -> (-74.9, -17.5)
extrude "Finestra_inserimento_SG90_Sinistra" cut sketch "Schizzo18 (2)" along normal blind 4 bodies 11 in component "04_Torretta_parte_fissa_azimut"
ref_plane "Piano di lavoro5" through (-40, 0, 0) normal (1, 0, 0) x (0, 1, 0) in component "04_Torretta_parte_fissa_azimut"
sketch "Schizzo19 (2)" plane through (-40, 0, 0) normal (1, 0, 0) x (0, 0, -1) in component "04_Torretta_parte_fissa_azimut"
  line L0 (-70.4, -8.15) -> (-74.9, -8.15)
  line L1 (-74.9, -8.15) -> (-74.9, -3.15)
  line L2 (-74.9, -3.15) -> (-70.4, -3.15)
  line L3 (-70.4, -3.15) -> (-70.4, -8.15)
extrude "Diramazione_cavo_5x4_5_SG90_Sinistra" cut sketch "Schizzo19 (2)" along normal blind 4 bodies 11 in component "04_Torretta_parte_fissa_azimut"
ref_plane "Piano di lavoro6" through (-40, 0, 0) normal (1, 0, 0) x (0, 1, 0) in component "04_Torretta_parte_fissa_azimut"
sketch "Schizzo20 (2)" plane through (-40, 0, 0) normal (1, 0, 0) x (0, 0, -1) in component "04_Torretta_parte_fissa_azimut"
  line L0 (-80.05, -23.7) -> (-82.95, -23.7)
  line L1 (-82.95, -23.7) -> (-82.95, -18.7)
  line L2 (-82.95, -18.7) -> (-80.05, -18.7)
  line L3 (-80.05, -18.7) -> (-80.05, -23.7)
extrude "Asola_M2_5_aletta_SG90_Sinistra_01" cut sketch "Schizzo20 (2)" along normal blind 4 bodies 11 in component "04_Torretta_parte_fissa_azimut"
ref_plane "Piano di lavoro7" through (-40, 0, 0) normal (1, 0, 0) x (0, 1, 0) in component "04_Torretta_parte_fissa_azimut"
sketch "Schizzo21 (2)" plane through (-40, 0, 0) normal (1, 0, 0) x (0, 0, -1) in component "04_Torretta_parte_fissa_azimut"
  line L0 (-80.05, 7.4) -> (-82.95, 7.4)
  line L1 (-82.95, 7.4) -> (-82.95, 12.4)
  line L2 (-82.95, 12.4) -> (-80.05, 12.4)
  line L3 (-80.05, 12.4) -> (-80.05, 7.4)
extrude "Asola_M2_5_aletta_SG90_Sinistra_02" cut sketch "Schizzo21 (2)" along normal blind 4 bodies 11 in component "04_Torretta_parte_fissa_azimut"
ref_plane "Piano di lavoro8" through (36, 0, 0) normal (1, 0, 0) x (0, 1, 0) in component "04_Torretta_parte_fissa_azimut"
sketch "Schizzo22 (2)" plane through (36, 0, 0) normal (1, 0, 0) x (0, 0, -1) in component "04_Torretta_parte_fissa_azimut"
  line L0 (-49.5, -35) -> (-99.5, -35)
  line L1 (-99.5, -35) -> (-99.5, 35)
  line L2 (-99.5, 35) -> (-49.5, 35)
  line L3 (-49.5, 35) -> (-49.5, -35)
extrude "Estrusione_Parete_fissa_Destra" add sketch "Schizzo22 (2)" along normal blind 4 bodies 11 in component "04_Torretta_parte_fissa_azimut"
ref_plane "Piano di lavoro9" through (36, 0, 0) normal (1, 0, 0) x (0, 1, 0) in component "04_Torretta_parte_fissa_azimut"
sketch "Schizzo23 (2)" plane through (36, 0, 0) normal (1, 0, 0) x (0, 0, -1) in component "04_Torretta_parte_fissa_azimut"
  line L0 (-74.9, -17.5) -> (-88.1, -17.5)
  line L1 (-88.1, -17.5) -> (-88.1, 6.2)
  line L2 (-88.1, 6.2) -> (-74.9, 6.2)
  line L3 (-74.9, 6.2) -> (-74.9, -17.5)
extrude "Finestra_inserimento_SG90_Destra" cut sketch "Schizzo23 (2)" along normal blind 4 bodies 11 in component "04_Torretta_parte_fissa_azimut"
ref_plane "Piano di lavoro10" through (36, 0, 0) normal (1, 0, 0) x (0, 1, 0) in component "04_Torretta_parte_fissa_azimut"
sketch "Schizzo24 (2)" plane through (36, 0, 0) normal (1, 0, 0) x (0, 0, -1) in component "04_Torretta_parte_fissa_azimut"
  line L0 (-70.4, -8.15) -> (-74.9, -8.15)
  line L1 (-74.9, -8.15) -> (-74.9, -3.15)
  line L2 (-74.9, -3.15) -> (-70.4, -3.15)
  line L3 (-70.4, -3.15) -> (-70.4, -8.15)
extrude "Diramazione_cavo_5x4_5_SG90_Destra" cut sketch "Schizzo24 (2)" along normal blind 4 bodies 11 in component "04_Torretta_parte_fissa_azimut"
ref_plane "Piano di lavoro11" through (36, 0, 0) normal (1, 0, 0) x (0, 1, 0) in component "04_Torretta_parte_fissa_azimut"
sketch "Schizzo25 (2)" plane through (36, 0, 0) normal (1, 0, 0) x (0, 0, -1) in component "04_Torretta_parte_fissa_azimut"
  line L0 (-80.05, -23.7) -> (-82.95, -23.7)
  line L1 (-82.95, -23.7) -> (-82.95, -18.7)
  line L2 (-82.95, -18.7) -> (-80.05, -18.7)
  line L3 (-80.05, -18.7) -> (-80.05, -23.7)
extrude "Asola_M2_5_aletta_SG90_Destra_01" cut sketch "Schizzo25 (2)" along normal blind 4 bodies 11 in component "04_Torretta_parte_fissa_azimut"
ref_plane "Piano di lavoro12" through (36, 0, 0) normal (1, 0, 0) x (0, 1, 0) in component "04_Torretta_parte_fissa_azimut"
sketch "Schizzo26 (2)" plane through (36, 0, 0) normal (1, 0, 0) x (0, 0, -1) in component "04_Torretta_parte_fissa_azimut"
  line L0 (-80.05, 7.4) -> (-82.95, 7.4)
  line L1 (-82.95, 7.4) -> (-82.95, 12.4)
  line L2 (-82.95, 12.4) -> (-80.05, 12.4)
  line L3 (-80.05, 12.4) -> (-80.05, 7.4)
extrude "Asola_M2_5_aletta_SG90_Destra_02" cut sketch "Schizzo26 (2)" along normal blind 4 bodies 11 in component "04_Torretta_parte_fissa_azimut"
ref_plane "Piano di lavoro13" through (0, 0, 72.4) normal (0, 0, 1) x (1, 0, 0) in component "04_Torretta_parte_fissa_azimut"
sketch "Schizzo27 (2)" plane through (0, 0, 72.4) normal (0, 0, 1) x (1, 0, 0) in component "04_Torretta_parte_fissa_azimut"
  line L0 (-63.5, -24.8) -> (-40, -24.8)
  line L1 (-40, -24.8) -> (-40, 13.5)
  line L2 (-40, 13.5) -> (-63.5, 13.5)
  line L3 (-63.5, 13.5) -> (-63.5, -24.8)
extrude "Estrusione_Slitta_SG90_Sinistra_ripiano_Inferiore" add sketch "Schizzo27 (2)" along normal blind 2.5 bodies 11 in component "04_Torretta_parte_fissa_azimut"
ref_plane "Piano di lavoro14" through (0, 0, 88.1) normal (0, 0, 1) x (1, 0, 0) in component "04_Torretta_parte_fissa_azimut"
sketch "Schizzo28 (2)" plane through (0, 0, 88.1) normal (0, 0, 1) x (1, 0, 0) in component "04_Torretta_parte_fissa_azimut"
  line L0 (-63.5, -24.8) -> (-40, -24.8)
  line L1 (-40, -24.8) -> (-40, 13.5)
  line L2 (-40, 13.5) -> (-63.5, 13.5)
  line L3 (-63.5, 13.5) -> (-63.5, -24.8)
extrude "Estrusione_Slitta_SG90_Sinistra_ripiano_Superiore" add sketch "Schizzo28 (2)" along normal blind 2.5 bodies 11 in component "04_Torretta_parte_fissa_azimut"
ref_plane "Piano di lavoro15" through (0, 0, 72.4) normal (0, 0, 1) x (1, 0, 0) in component "04_Torretta_parte_fissa_azimut"
sketch "Schizzo29 (2)" plane through (0, 0, 72.4) normal (0, 0, 1) x (1, 0, 0) in component "04_Torretta_parte_fissa_azimut"
  line L0 (-63.5, -8.15) -> (-61.5, -8.15)
  line L1 (-61.5, -8.15) -> (-61.5, -3.15)
  line L2 (-61.5, -3.15) -> (-63.5, -3.15)
  line L3 (-63.5, -3.15) -> (-63.5, -8.15)
extrude "Uscita_cavo_5x2_SG90_Sinistra" cut sketch "Schizzo29 (2)" along normal blind 2.5 bodies 11 in component "04_Torretta_parte_fissa_azimut"
ref_plane "Piano di lavoro16" through (-63.5, 0, 0) normal (1, 0, 0) x (0, 1, 0) in component "04_Torretta_parte_fissa_azimut"
sketch "Schizzo30 (2)" plane through (-63.5, 0, 0) normal (1, 0, 0) x (0, 0, -1) in component "04_Torretta_parte_fissa_azimut"
  line L0 (-74.9, -24.8) -> (-88.1, -24.8)
  line L1 (-88.1, -24.8) -> (-88.1, -22.3)
  line L2 (-88.1, -22.3) -> (-74.9, -22.3)
  line L3 (-74.9, -22.3) -> (-74.9, -24.8)